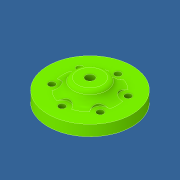
# Autodesk Inventor part: GripperMountPlatehock
Saved by Autodesk Inventor 2016 (Build 200138000, 138)
## iProperties
Created: 2015-09-10
Part Number: GripperMountPlatehock
Material: ABS-Kunststoff
Document SubType Name: Modeling
Designer: 4ndreas
Density: 1.06 g/cm^3
Appearance: Glatt - grün
Mass: 7.0775 g
Surface Area: 34.9537 cm^2
Volume: 6.67689 cm^3
Author: 4ndreas
Autodesk Inventor part; units mm, degrees
ref_plane "YZ Plane" through (0, 0, 0) normal (1, 0, 0) x (0, 1, 0)
ref_plane "XZ Plane" through (0, 0, 0) normal (0, 1, 0) x (-1, 0, 0)
ref_plane "XY Plane" through (0, 0, 0) normal (0, 0, 1) x (1, 0, 0)
sketch "Skizze1" plane through (0, 0, 0) normal (0, 0, 1) x (1, 0, 0)
  circle A0 centre (-11.2583, 6.5) radius 1.5 projected
  circle A1 centre (-11.2583, -6.5) radius 1.5 projected
  circle A2 centre (0, -13) radius 1.5 projected
  circle A3 centre (11.2583, -6.5) radius 1.5 projected
  circle A4 centre (11.2583, 6.5) radius 1.5 projected
  circle A5 centre (0, 13) radius 1.5 projected
  arc A6 (14.3761, 1.8914) -> (11.9393, 3.5783) centre (12.3932, 1.6305) ccw projected
  arc A7 (14.3761, -1.8914) -> (14.3761, 1.8914) centre (0, 0) ccw projected
  arc A8 (11.9393, -3.5783) -> (14.3761, -1.8914) centre (12.3932, -1.6305) ccw projected
  arc A9 (11.9393, -3.5783) -> (9.0685, -8.5505) centre (11.2583, -6.5) ccw projected
  arc A10 (8.826, -11.5044) -> (9.0685, -8.5505) centre (7.6087, -9.9176) ccw projected
  arc A11 (5.5501, -13.3958) -> (8.826, -11.5044) centre (0, 0) ccw projected
  arc A12 (2.8707, -12.1288) -> (5.5501, -13.3958) centre (4.7846, -11.5481) ccw projected
  arc A13 (2.8707, -12.1288) -> (-2.8707, -12.1288) centre (0, -13) ccw projected
  arc A14 (-5.5501, -13.3958) -> (-2.8707, -12.1288) centre (-4.7846, -11.5481) ccw projected
  arc A15 (-8.826, -11.5044) -> (-5.5501, -13.3958) centre (0, 0) ccw projected
  arc A16 (-9.0685, -8.5505) -> (-8.826, -11.5044) centre (-7.6087, -9.9176) ccw projected
  arc A17 (-9.0685, -8.5505) -> (-11.9393, -3.5783) centre (-11.2583, -6.5) ccw projected
  arc A18 (-14.3761, -1.8914) -> (-11.9393, -3.5783) centre (-12.3932, -1.6305) ccw projected
  arc A19 (-14.3761, 1.8914) -> (-14.3761, -1.8914) centre (0, 0) ccw projected
  arc A20 (-11.9393, 3.5783) -> (-14.3761, 1.8914) centre (-12.3932, 1.6305) ccw projected
  arc A21 (-11.9393, 3.5783) -> (-9.0685, 8.5505) centre (-11.2583, 6.5) ccw projected
  arc A22 (-8.826, 11.5044) -> (-9.0685, 8.5505) centre (-7.6087, 9.9176) ccw projected
  arc A23 (-5.5501, 13.3958) -> (-8.826, 11.5044) centre (0, 0) ccw projected
  arc A24 (-2.8707, 12.1288) -> (-5.5501, 13.3958) centre (-4.7846, 11.5481) ccw projected
  arc A25 (-2.8707, 12.1288) -> (2.8707, 12.1288) centre (0, 13) ccw projected
  arc A26 (5.5501, 13.3958) -> (2.8707, 12.1288) centre (4.7846, 11.5481) ccw projected
  arc A27 (8.826, 11.5044) -> (5.5501, 13.3958) centre (0, 0) ccw projected
  arc A28 (9.0685, 8.5505) -> (8.826, 11.5044) centre (7.6087, 9.9176) ccw projected
  arc A29 (9.0685, 8.5505) -> (11.9393, 3.5783) centre (11.2583, 6.5) ccw projected
  circle A30 centre (0, 0) radius 17.5 projected
  circle A31 centre (0, 0) radius 19.5
  point P0 (0, 0)
  dimension "d0" = 39
  constraints: 1 centre point, 1 coincident
  measures "d0" diameter of A31
extrude "Extrusion1" add sketch "Skizze1" along normal blind 5 contours A7 A8 A9 A10 A11 A12 A13 A14 A15 A16 A17 A18 A19 A20 A21 A22 A23 A24 A25 A26 A27 A28 A29 A6 | A30 | A31
sketch "Skizze2" plane through (0, 0, 5) normal (0, 0, 1) x (1, 0, 0)
  circle A0 centre (0, 0) radius 7.5
  dimension "d3" = 15
  constraints: 1 centre point, 1 coincident
  measures "d3" diameter of A0
extrude "Extrusion2" add sketch "Skizze2" along normal blind 5
sketch "Skizze6" plane through (0, 0, 5) normal (0, 0, 1) x (1, 0, 0)
  circle A0 centre (0, 0) radius 7.5 projected
  circle A1 centre (0, 13) radius 1.5 projected
  circle A2 centre (11.2583, 6.5) radius 1.5 projected
  circle A3 centre (11.2583, -6.5) radius 1.5 projected
  circle A4 centre (0, -13) radius 1.5 projected
  circle A5 centre (-11.2583, -6.5) radius 1.5 projected
  circle A6 centre (-11.2583, 6.5) radius 1.5 projected
  circle A7 centre (0, 0) radius 19.5 projected
  circle A8 centre (11.2583, 6.5) radius 3.5
  dimension "d20" = 7
  constraints: 1 centre point
  measures "d20" diameter of A8
fillet "Rundung1" radius 5 1 edges at (-7.5, 0, 5)
fillet "Rundung2" radius 2 1 edges at (-7.5, 0, 10)
sketch "Skizze3" plane through (0, 0, 0) normal (0, 0, -1) x (-1, 0, 0)
  line L0 (0, -4.0415) -> (-3.5, -2.0207)
  line L1 (-3.5, -2.0207) -> (-3.5, 2.0207)
  line L2 (-3.5, 2.0207) -> (0, 4.0415)
  line L3 (0, 4.0415) -> (3.5, 2.0207)
  line L4 (3.5, 2.0207) -> (3.5, -2.0207)
  line L5 (3.5, -2.0207) -> (0, -4.0415)
  point P0 (0, 0)
  point P1 (0, 0)
  dimension "d8" = 7
  constraints: 12 end point, 1 coincident, 1 vertical, 13 other
  measures "d8" distance between parallel lines of L1 L4
sketch "Skizze4" plane through (0, 0, 10) normal (0, 0, 1) x (1, 0, 0)
  point P0 (0, 0)
hole "Bohrung1" at (0, 0, 10) direction (0, 0, -1) diameter 4 end through all
extrude "Extrusion3" cut sketch "Skizze3" against normal blind 3
sketch "Skizze5" plane through (0, 0, 3) normal (0, 0, -1) x (-1, 0, 0)
  circle A0 centre (0, 0) radius 2 projected
  circle A1 centre (0, 0) radius 2 projected
extrude "Extrusion4" add sketch "Skizze5" against normal blind 0.2
extrude "Extrusion5" cut sketch "Skizze6" along normal blind 10 contours A2 | A8
pattern_circular "Runde Anordnung1" count 6 over 360 about axis through (0, 0, -46.0535) along (0, 0, 1) of "Extrusion5"
